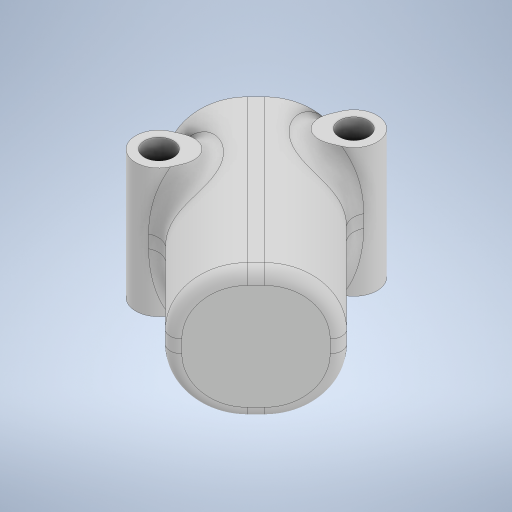
# Autodesk Inventor part: 4700uF cap holder
Saved by Autodesk Inventor 2023 (Build 270158000, 158)
## iProperties
Created: 2023-01-22
Part Number: 4700uF cap holder
Material: Generic
Document SubType Name: Modeling
Designer: Steven
Density: 1 g/cm^3
Appearance: Default
Author: Steven
Autodesk Inventor part; units mm, degrees
ref_plane "YZ Plane" through (0, 0, 0) normal (1, 0, 0) x (0, 1, 0)
ref_plane "XZ Plane" through (0, 0, 0) normal (0, 1, 0) x (-1, 0, 0)
ref_plane "XY Plane" through (0, 0, 0) normal (0, 0, 1) x (1, 0, 0)
sketch "Sketch1" plane through (0, 0, 0) normal (0, 1, 0) x (-1, 0, 0)
  circle A0 centre (0, 0) radius 2.5
  circle A1 centre (13.759351, 19.850542) radius 2.5
  line L0 (-17.951707, 22.037643) -> (6.79703, -2.711095) construction
  line L1 (5.382817, -4.125308) -> (20.993387, 11.485262)
  line L2 (-5.169564, 34.819786) -> (19.579173, 10.071048) construction
  line L3 (-17.995307, 21.994043) -> (-5.125964, 34.863386) construction
  arc A2 (15.965023, 16.513626) -> (10.422434, 22.056214) centre (13.759351, 19.850542) ccw
  arc A3 (-2.128902, 3.386411) -> (3.386411, -2.128902) centre (0, 0) ccw
  line L4 (-5.169564, 37.648213) -> (11.518894, 20.959755)
  line L5 (-20.780134, 22.037643) -> (-1.023416, 2.280925)
  line L6 (-20.780134, 22.037643) -> (-5.169564, 37.648213)
  line L7 (14.868564, 17.610085) -> (20.993387, 11.485262)
  line L8 (11.518894, 20.959755) -> (14.868564, 17.610085)
  line L9 (2.280925, -1.023416) -> (5.382817, -4.125308)
  line L10 (-1.023416, 2.280925) -> (2.280925, -1.023416)
  arc A4 (13.799478, 15.850743) -> (15.965023, 16.513626) centre (13.759351, 19.850542) ccw
  arc A5 (10.422434, 22.056214) -> (13.799478, 15.850743) centre (13.759351, 19.850542) ccw
  arc A6 (0.08688, 3.999056) -> (-2.128902, 3.386411) centre (0, 0) ccw
  arc A7 (3.386411, -2.128902) -> (0.08688, 3.999056) centre (0, 0) ccw
  dimension "d0" = 8
  dimension "d1" = 8
  dimension "d2" = 2
  dimension "d3" = 2
  dimension "d4" = 2
  constraints: 22 end point, 16 point on circle, 8 centre point, 7 parallel, 6 point on line, 2 coincident, 10 other
  measures "d0" diameter of A2
  measures "d1" diameter of A3
  measures "d2" distance between parallel lines of L2 L4
  measures "d3" distance between parallel lines of L0 L5
  measures "d4" distance between parallel lines of L3 L6
extrude "Extrusion1" add sketch "Sketch1" along normal blind 22.2 contours A0 L10 | A0 L5 A6 A7 L9 | L5 L6 L4 A5 A4 L7 L1 L9 A7 A6 | L4 A1 L7 A4 A5 | L8 A1 picked at (1.030494, 0.985498) picked at (12.323251, 18.602841)
fillet "Fillet1" radius 10 12 edges at (-3.8319, 22.2, -2.5744) (-0.6288, 22.2, 0.6288) (10.9018, 22.2, 12.1593) (-3.1747, 22.2, 29.304) (-13.1937, 22.2, 19.2849) (-17.931, 22.2, 14.5477) (-3.1747, 0, 29.304) (-13.1937, 0, 19.2849) (-17.931, 0, 14.5477) (-3.8319, 0, -2.5744) (-0.6288, 0, 0.6288) (10.9018, 0, 12.1593)
extrude "Extrusion2" add sketch "Sketch1" along normal blind 22.2 contours A0 L10 | A0 L5 A6 A7 L9 | L10 A0 | A0 L9 A3 L5 | A2 L7 A1 L4 | L4 A1 L7 A4 A5 | L8 A1 | A1 L8
extrude "Extrusion3" cut sketch "Sketch1" along normal blind 22.2 contours A0 L10 | L10 A0 | L8 A1 | A1 L8
sketch "Sketch2" plane through (-20.993387, 10, 11.485262) normal (-0.7071068, 0, -0.7071068) x (-0.7071068, 0, 0.7071068)
  arc A0 (-22.07668, 0) -> (-12.07668, -10) centre (-12.07668, 0) ccw
  line L0 (-12.07668, -10) -> (-10, -10)
  arc A1 (-10, -10) -> (0, 0) centre (-10, 0) ccw
  line L1 (0, 0) -> (0, 2.2)
  arc A2 (0, 2.2) -> (-10, 12.2) centre (-10, 2.2) ccw
  line L2 (-12.07668, 12.2) -> (-10, 12.2)
  arc A3 (-12.07668, 12.2) -> (-22.07668, 2.2) centre (-12.07668, 2.2) ccw
  line L3 (-22.07668, 0) -> (-22.07668, 2.2)
  line L4 (-12.07668, 2.2) -> (-10, 0) construction
  point P0 (-22.965873, -10)
  point P1 (-11.03834, 1.1)
  constraints: 2 end point, 1 midpoint
hole "Hole1" at (-13.188102, 11.1, 3.679977) direction (0.7071068, 0, 0.7071068) diameter 18.4 depth 35
fillet "Fillet2" radius 2 8 edges at (20.7801, 11.1, 22.0376) (18.7091, 2.9289, 24.1087) (12.9748, 0, 29.8429) (7.2406, 2.9289, 35.5771) (5.1696, 11.1, 37.6482) (7.2406, 19.2711, 35.5771) (12.9748, 22.2, 29.8429) (18.7091, 19.2711, 24.1087)
fillet "Fillet3" radius 3 16 edges at (2.1289, 11.1, 3.3864) (-3.6923, 15.7034, -1.5385) (-2.8284, 19.4484, 2.8284) (1.5382, 15.7041, 3.6924) (-3.3864, 11.1, -2.1289) (1.5382, 6.4959, 3.6924) (-2.8284, 2.7516, 2.8284) (-3.6923, 6.4966, -1.5385) (-15.965, 11.1, 16.5136) (-10.0981, 15.7462, 21.4615) (-15.3701, 15.7466, 16.1892) (-10.9309, 19.5322, 17.0221) (-10.4224, 11.1, 22.0562) (-10.0981, 6.4538, 21.4615) (-15.3701, 6.4534, 16.1892) (-10.9309, 2.6678, 17.0221)
body "Solid1"
